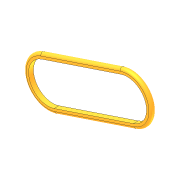
# Autodesk Inventor part: Belt_HorizontalIntake_Front
Saved by Autodesk Inventor 2012 (Build 160160000, 160)
## iProperties
Created: 2012-01-22
Part Number: Belt_HorizontalIntake_Front
Material: High Density Polyethylene
Document SubType Name: Modeling
Designer: JesseK
Density: 0.952 g/cm^3
Mass: 5.50632 g
Surface Area: 48.4603 cm^2
Volume: 5.78395 cm^3
Author: JesseK
Autodesk Inventor part; units mm, degrees
ref_plane "YZ Plane" through (0, 0, 0) normal (1, 0, 0) x (0, 1, 0)
ref_plane "XZ Plane" through (0, 0, 0) normal (0, 1, 0) x (-1, 0, 0)
ref_plane "XY Plane" through (0, 0, 0) normal (0, 0, 1) x (1, 0, 0)
sketch "Sketch1" plane through (0, 0, 0) normal (0, 0, 1) x (1, 0, 0)
  arc A0 (-6.0433, 18.066) -> (6.0433, -18.066) centre (0, 0) ccw
  arc A1 (84.3294, 8.1215) -> (72.2428, 44.2536) centre (78.2861, 26.1876) ccw
  line L0 (-6.0433, 18.066) -> (72.2428, 44.2536)
  line L1 (84.3294, 8.1215) -> (6.0433, -18.066)
  arc A2 (-7.5541, 22.5825) -> (7.5541, -22.5825) centre (0, 0) ccw
  arc A3 (85.8402, 3.605) -> (70.732, 48.7701) centre (78.2861, 26.1876) ccw
  line L2 (7.5541, -22.5825) -> (85.8402, 3.605)
  line L3 (70.732, 48.7701) -> (-7.5541, 22.5825)
  dimension "d0" = 19.05
  dimension "d1" = 82.55
  dimension "d2" = 4.7625
  constraints: 8 end point, 8 point on circle, 7 tangent, 4 centre point, 3 coincident, 2 parallel, 1 equal radius
  measures "d0" radius of A0
  measures "d1" distance of L0.start L0.end
  measures "d2" distance between parallel lines of L0 L3
extrude "Extrusion1" add sketch "Sketch1" along normal blind 4.7625
fillet "Fillet1" radius 2.3813 8 edges at (-22.5825, -7.5541, 0) (46.6972, -9.4887, 0) (100.8686, 33.7417, 0) (31.5889, 35.6763, 0) (100.8686, 33.7417, 4.7625) (46.6972, -9.4887, 4.7625) (-22.5825, -7.5541, 4.7625) (31.5889, 35.6763, 4.7625)
body "Solid1"
